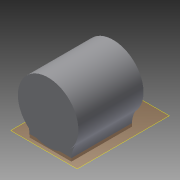
# Autodesk Inventor part: Motor4
Saved by Autodesk Inventor 2015 (Build 190159000, 159)
## iProperties
Created: 2016-02-24
Part Number: Motor4
Material: Generic
Document SubType Name: Modeling
Designer: jonesdm
Density: 1 g/cm^3
Appearance: Default
Author: jonesdm
Autodesk Inventor part; units mm, degrees
ref_plane "YZ Plane" through (0, 0, 0) normal (1, 0, 0) x (0, 1, 0)
ref_plane "XY Plane" through (0, 0, 0) normal (0, 0, 1) x (1, 0, 0)
sketch "Sketch1" plane through (0, 0, 0) normal (0, 0, 1) x (1, 0, 0)
  circle A0 centre (0, 0) radius 7.9375
  line L0 (-2.4257, 7.5578) -> (-2.4257, 10.0978)
  line L1 (-2.4257, 10.0978) -> (2.4257, 10.0978)
  line L2 (2.4257, 10.0978) -> (2.4257, 7.5578)
  point P0 (0, 10.0978)
  dimension "d0" = 15.875
  dimension "d1" = 2.54
  dimension "d2" = 4.8514
  constraints: 6 end point, 2 point on circle, 1 centre point, 1 coincident, 1 horizontal, 1 midpoint, 1 perpendicular, 1 vertical, 1 vertical alignment
  measures "d0" diameter of A0
  measures "d1" distance of L1.end L2.end
  measures "d2" distance of L0.end L1.end
extrude "Extrusion1" add sketch "Sketch1" along normal blind 50.8
sketch "Sketch2" plane through (0, 0, 50.8) normal (0, 0, 1) x (1, 0, 0)
  circle A0 centre (0, 0) radius 82.55
  dimension "d5" = 165.1
  constraints: 1 centre point, 1 coincident
  measures "d5" diameter of A0
extrude "Extrusion2" add sketch "Sketch2" along normal blind 177.8
sketch "Sketch3" plane through (0, 0, 50.8) normal (0, 0, -1) x (-1, 0, 0)
  circle A0 centre (0, 0) radius 73.025
  arc A1 (-2.4257, 7.5578) -> (2.4257, 7.5578) centre (0, 0) ccw projected
  line L0 (0, 0) -> (51.6365, 51.6365)
  line L1 (0, 0) -> (73.025, 0) construction
  line L2 (0, 0) -> (51.6365, -51.6365)
  line L3 (0, 0) -> (73.025, 0) construction
  line L4 (0, 0) -> (-51.6365, 51.6365)
  line L5 (0, 0) -> (73.025, 0) construction
  line L6 (0, 0) -> (-51.6365, -51.6365)
  line L7 (0, 0) -> (73.025, 0) construction
  dimension "d8" = 146.05
  dimension "d9" = 45
  dimension "d10" = 45
  dimension "d11" = 135
  dimension "d12" = 135
  constraints: 16 end point, 5 coincident, 4 equal length, 4 horizontal, 4 point on circle, 1 centre point
  measures "d8" diameter of A0
  measures "d9" angle of L1 L0
  measures "d10" angle of L2 L3
  measures "d11" angle of L5 L4
  measures "d12" angle of L6 L7
hole "Hole1" at (51.6365, 51.6365, 50.8) at (-51.6365, 51.6365, 50.8) at (-51.6365, -51.6365, 50.8) at (51.6365, -51.6365, 50.8) direction (0, 0, 1) diameter 4.9784 depth 19.05 tip angle 118 thread size "1/4-20 UNC" class "2B" standard "ANSI Unified Screw Threads"
ref_plane "Work Plane1" through (0, -82.55, 50.8) normal (0, 1, 0) x (-1, 0, 0)
sketch "Sketch4" plane through (0, -82.55, 50.8) normal (0, 1, 0) x (-1, 0, 0)
  line L0 (82.55, 177.8) -> (-82.55, 177.8) projected
  line L1 (-82.55, 0) -> (82.55, 0) projected
  line L2 (82.55, 0) -> (82.55, 177.8) projected
  line L3 (-82.55, 0) -> (-82.55, 177.8) projected
  line L4 (-57.15, 6.35) -> (57.15, 6.35)
  line L5 (57.15, 6.35) -> (57.15, 171.45)
  line L6 (57.15, 171.45) -> (-57.15, 171.45)
  line L7 (-57.15, 171.45) -> (-57.15, 6.35)
  point P0 (0, -50.8)
  point P1 (0, 6.35)
  dimension "d20" = 165.1
  dimension "d21" = 6.35
  dimension "d22" = 114.3
  constraints: 8 end point, 2 parallel, 1 horizontal, 1 midpoint, 1 perpendicular, 1 vertical alignment
  measures "d20" distance of L4.end L5.end
  measures "d21" distance between parallel lines of L1 L4
  measures "d22" distance of L4.start L4.end
extrude "Extrusion3" add sketch "Sketch4" along normal blind 25.4 and the other way blind 8.4074 contours L7 L6 L5 L4
fillet "Fillet1" radius 76.2 1 edges at (-57.15, -59.5683, 139.7)
fillet "Fillet2" radius 76.2 1 edges at (57.15, -59.5683, 139.7)
equation "\"d3\" = ShaftL"
equation "\"d5\" = MotoD"
equation "\"d6\" = MotoL"
equation "\"ShaftL\" = 50.8"
equation "\"MotoD\" = 165.1"
equation "\"MotoL\" = 177.8"
body "Solid1"
